Autodesk Fusion 360 part; units mm, degrees
(part 4 of 5)
  spline S14 degree 5 poles (-104.9129, -27.728) (-104.9107, -27.7405) (-104.9058, -27.7653) (-104.8975, -27.8023) (-104.8848, -27.8513) (-104.8664, -27.9119) (-104.8463, -27.9721) (-104.8251, -28.0321) (-104.8033, -28.0919) (-104.7812, -28.1516) (-104.7586, -28.2113) (-104.7355, -28.2708) (-104.7117, -28.3301) (-104.687, -28.3892) (-104.6615, -28.4481) (-104.6353, -28.5068) (-104.6083, -28.5653) (-104.5809, -28.6236) (-104.5529, -28.6818) (-104.5245, -28.7398) (-104.4956, -28.7977) (-104.4663, -28.8555) (-104.4364, -28.9131) (-104.4061, -28.9706) (-104.3752, -29.0279) (-104.3439, -29.085) (-104.312, -29.142) (-104.2798, -29.1989) (-104.2471, -29.2556) (-104.214, -29.3121) (-104.1805, -29.3686) (-104.1466, -29.4249) (-104.1123, -29.481) (-104.0776, -29.537) (-104.0425, -29.5929) (-104.0069, -29.6486) (-103.971, -29.7042) (-103.9348, -29.7596) (-103.8981, -29.8149) (-103.8611, -29.8701) (-103.8237, -29.9251) (-103.786, -29.98) (-103.7479, -30.0347) (-103.7094, -30.0893) (-103.6707, -30.1438) (-103.6315, -30.1981) (-103.592, -30.2523) (-103.5522, -30.3063) (-103.5121, -30.3603) (-103.4716, -30.414) (-103.4308, -30.4677) (-103.3896, -30.5212) (-103.3482, -30.5745) (-103.3064, -30.6277) (-103.2643, -30.6808) (-103.2219, -30.7337) (-103.1792, -30.7865) (-103.1362, -30.8392) (-103.0928, -30.8917) (-103.0492, -30.9441) (-103.0053, -30.9963) (-102.9611, -31.0484) (-102.9165, -31.1004) (-102.8717, -31.1522) (-102.8266, -31.2039) (-102.7812, -31.2554) (-102.7355, -31.3068) (-102.6896, -31.3581) (-102.6433, -31.4092) (-102.5968, -31.4601) (-102.55, -31.511) (-102.5123, -31.5515) (-102.4839, -31.5819) (-102.4649, -31.6021) (-102.4554, -31.6122) knots 0 0 0 0 0 0 0.01428571 0.02857143 0.04285714 0.05714286 0.07142857 0.08571429 0.1 0.11428571 0.12857143 0.14285714 0.15714286 0.17142857 0.18571429 0.2 0.21428571 0.22857143 0.24285714 0.25714286 0.27142857 0.28571429 0.3 0.31428571 0.32857143 0.34285714 0.35714286 0.37142857 0.38571429 0.4 0.41428571 0.42857143 0.44285714 0.45714286 0.47142857 0.48571429 0.5 0.51428571 0.52857143 0.54285714 0.55714286 0.57142857 0.58571429 0.6 0.61428571 0.62857143 0.64285714 0.65714286 0.67142857 0.68571429 0.7 0.71428571 0.72857143 0.74285714 0.75714286 0.77142857 0.78571429 0.8 0.81428571 0.82857143 0.84285714 0.85714286 0.87142857 0.88571429 0.9 0.91428571 0.92857143 0.94285714 0.95714286 0.97142857 0.98571429 1 1 1 1 1 1
  arc A30 (-102.4554, -31.6122) -> (-100.7277, -31.1492) centre (-110, 0) ccw
  spline S15 degree 5 poles (-100.7277, -31.1492) (-100.7245, -31.1357) (-100.7182, -31.1088) (-100.7088, -31.0683) (-100.6964, -31.0143) (-100.6813, -30.9469) (-100.6665, -30.8795) (-100.652, -30.8121) (-100.6378, -30.7447) (-100.624, -30.6774) (-100.6104, -30.61) (-100.5972, -30.5427) (-100.5843, -30.4755) (-100.5717, -30.4082) (-100.5594, -30.341) (-100.5475, -30.2738) (-100.5359, -30.2066) (-100.5247, -30.1394) (-100.5137, -30.0723) (-100.5031, -30.0052) (-100.4929, -29.9382) (-100.483, -29.8712) (-100.4734, -29.8042) (-100.4642, -29.7373) (-100.4553, -29.6704) (-100.4468, -29.6035) (-100.4386, -29.5367) (-100.4308, -29.47) (-100.4233, -29.4032) (-100.4162, -29.3366) (-100.4095, -29.27) (-100.4031, -29.2034) (-100.3971, -29.1369) (-100.3915, -29.0704) (-100.3863, -29.004) (-100.3814, -28.9377) (-100.3769, -28.8714) (-100.3728, -28.8052) (-100.3691, -28.739) (-100.3658, -28.673) (-100.3629, -28.607) (-100.3605, -28.541) (-100.3584, -28.4752) (-100.3568, -28.4094) (-100.3555, -28.3437) (-100.3547, -28.2781) (-100.3544, -28.2125) (-100.3544, -28.1471) (-100.3549, -28.0817) (-100.3559, -28.0164) (-100.3573, -27.9513) (-100.3592, -27.8862) (-100.3616, -27.8213) (-100.3646, -27.7565) (-100.3681, -27.6918) (-100.372, -27.6272) (-100.3765, -27.5627) (-100.3813, -27.4983) (-100.3867, -27.4341) (-100.3926, -27.37) (-100.3992, -27.306) (-100.4066, -27.2423) (-100.4148, -27.1788) (-100.4238, -27.1155) (-100.4335, -27.0524) (-100.4438, -26.9894) (-100.4545, -26.9266) (-100.4656, -26.8639) (-100.4772, -26.8014) (-100.4899, -26.7392) (-100.5043, -26.6775) (-100.5177, -26.6288) (-100.5291, -26.5926) (-100.5373, -26.5686) (-100.5415, -26.5567) knots -1 -1 -1 -1 -1 -1 -0.98571429 -0.97142857 -0.95714286 -0.94285714 -0.92857143 -0.91428571 -0.9 -0.88571429 -0.87142857 -0.85714286 -0.84285714 -0.82857143 -0.81428571 -0.8 -0.78571429 -0.77142857 -0.75714286 -0.74285714 -0.72857143 -0.71428571 -0.7 -0.68571429 -0.67142857 -0.65714286 -0.64285714 -0.62857143 -0.61428571 -0.6 -0.58571429 -0.57142857 -0.55714286 -0.54285714 -0.52857143 -0.51428571 -0.5 -0.48571429 -0.47142857 -0.45714286 -0.44285714 -0.42857143 -0.41428571 -0.4 -0.38571429 -0.37142857 -0.35714286 -0.34285714 -0.32857143 -0.31428571 -0.3 -0.28571429 -0.27142857 -0.25714286 -0.24285714 -0.22857143 -0.21428571 -0.2 -0.18571429 -0.17142857 -0.15714286 -0.14285714 -0.12857143 -0.11428571 -0.1 -0.08571429 -0.07142857 -0.05714286 -0.04285714 -0.02857143 -0.01428571 0 0 0 0 0 0
  line L15 (-100.5415, -26.5567) -> (-100.5754, -26.4615)
  arc A31 (-100.0022, -25.1964) -> (-100.5754, -26.4615) centre (-99.6334, -26.1259) ccw
  arc A32 (-100.0022, -25.1964) -> (-99.2529, -24.8861) centre (-110, 0) ccw
  arc A33 (-97.9531, -25.3753) -> (-99.2529, -24.8861) centre (-98.8565, -25.8041) ccw
  line L16 (-97.9531, -25.3753) -> (-97.9097, -25.4666)
  spline S16 degree 5 poles (-97.9097, -25.4666) (-97.9043, -25.478) (-97.8932, -25.5007) (-97.8756, -25.5344) (-97.8506, -25.5783) (-97.8172, -25.6321) (-97.7822, -25.6851) (-97.7462, -25.7375) (-97.7097, -25.7897) (-97.6728, -25.8417) (-97.6356, -25.8934) (-97.5979, -25.9449) (-97.5595, -25.9961) (-97.5204, -26.0468) (-97.4805, -26.0971) (-97.44, -26.1469) (-97.3988, -26.1965) (-97.3572, -26.2457) (-97.3151, -26.2946) (-97.2726, -26.3434) (-97.2298, -26.3918) (-97.1865, -26.44) (-97.1427, -26.488) (-97.0985, -26.5356) (-97.0539, -26.583) (-97.0088, -26.6301) (-96.9633, -26.6769) (-96.9175, -26.7234) (-96.8712, -26.7698) (-96.8246, -26.8158) (-96.7777, -26.8617) (-96.7303, -26.9073) (-96.6827, -26.9526) (-96.6346, -26.9977) (-96.5863, -27.0426) (-96.5375, -27.0872) (-96.4885, -27.1316) (-96.4391, -27.1758) (-96.3894, -27.2197) (-96.3393, -27.2634) (-96.289, -27.3069) (-96.2383, -27.3501) (-96.1874, -27.3931) (-96.1361, -27.4359) (-96.0845, -27.4785) (-96.0327, -27.5208) (-95.9805, -27.563) (-95.9281, -27.6049) (-95.8753, -27.6466) (-95.8223, -27.688) (-95.769, -27.7293) (-95.7154, -27.7703) (-95.6616, -27.8111) (-95.6074, -27.8517) (-95.5531, -27.892) (-95.4984, -27.9322) (-95.4435, -27.9721) (-95.3883, -28.0119) (-95.3328, -28.0514) (-95.2771, -28.0907) (-95.2212, -28.1298) (-95.165, -28.1687) (-95.1085, -28.2073) (-95.0518, -28.2458) (-94.9949, -28.284) (-94.9377, -28.322) (-94.8803, -28.3599) (-94.8226, -28.3975) (-94.7647, -28.4349) (-94.7065, -28.4721) (-94.6482, -28.509) (-94.6013, -28.5385) (-94.566, -28.5604) (-94.5425, -28.575) (-94.5307, -28.5823) knots 0 0 0 0 0 0 0.01428571 0.02857143 0.04285714 0.05714286 0.07142857 0.08571429 0.1 0.11428571 0.12857143 0.14285714 0.15714286 0.17142857 0.18571429 0.2 0.21428571 0.22857143 0.24285714 0.25714286 0.27142857 0.28571429 0.3 0.31428571 0.32857143 0.34285714 0.35714286 0.37142857 0.38571429 0.4 0.41428571 0.42857143 0.44285714 0.45714286 0.47142857 0.48571429 0.5 0.51428571 0.52857143 0.54285714 0.55714286 0.57142857 0.58571429 0.6 0.61428571 0.62857143 0.64285714 0.65714286 0.67142857 0.68571429 0.7 0.71428571 0.72857143 0.74285714 0.75714286 0.77142857 0.78571429 0.8 0.81428571 0.82857143 0.84285714 0.85714286 0.87142857 0.88571429 0.9 0.91428571 0.92857143 0.94285714 0.95714286 0.97142857 0.98571429 1 1 1 1 1 1
  arc A34 (-94.5307, -28.5823) -> (-92.9816, -27.688) centre (-110, 0) ccw
  spline S17 degree 5 poles (-92.9816, -27.688) (-92.9821, -27.6741) (-92.9829, -27.6464) (-92.9843, -27.6049) (-92.9864, -27.5496) (-92.9892, -27.4806) (-92.9923, -27.4116) (-92.9958, -27.3428) (-92.9995, -27.274) (-93.0035, -27.2054) (-93.0079, -27.1368) (-93.0125, -27.0684) (-93.0175, -27.0001) (-93.0227, -26.9318) (-93.0283, -26.8637) (-93.0342, -26.7957) (-93.0404, -26.7278) (-93.0469, -26.6601) (-93.0537, -26.5924) (-93.0608, -26.5249) (-93.0683, -26.4574) (-93.076, -26.3902) (-93.0841, -26.323) (-93.0925, -26.2559) (-93.1013, -26.189) (-93.1103, -26.1223) (-93.1197, -26.0556) (-93.1295, -25.9891) (-93.1395, -25.9227) (-93.1499, -25.8565) (-93.1607, -25.7904) (-93.1717, -25.7245) (-93.1832, -25.6587) (-93.1949, -25.593) (-93.2071, -25.5275) (-93.2195, -25.4622) (-93.2324, -25.397) (-93.2455, -25.332) (-93.2591, -25.2671) (-93.273, -25.2025) (-93.2873, -25.1379) (-93.302, -25.0736) (-93.317, -25.0095) (-93.3324, -24.9455) (-93.3483, -24.8817) (-93.3645, -24.8181) (-93.3811, -24.7547) (-93.3981, -24.6915) (-93.4155, -24.6285) (-93.4333, -24.5657) (-93.4515, -24.5031) (-93.4702, -24.4408) (-93.4894, -24.3787) (-93.509, -24.3169) (-93.5291, -24.2553) (-93.5497, -24.1939) (-93.5706, -24.1328) (-93.592, -24.0718) (-93.6138, -24.0112) (-93.6361, -23.9508) (-93.659, -23.8907) (-93.6826, -23.8311) (-93.707, -23.7718) (-93.7321, -23.713) (-93.7578, -23.6546) (-93.7841, -23.5965) (-93.8106, -23.5386) (-93.8375, -23.4809) (-93.865, -23.4235) (-93.8933, -23.3667) (-93.9232, -23.3108) (-93.9488, -23.2672) (-93.9691, -23.2352) (-93.9832, -23.2142) (-93.9904, -23.2037) knots -1 -1 -1 -1 -1 -1 -0.98571429 -0.97142857 -0.95714286 -0.94285714 -0.92857143 -0.91428571 -0.9 -0.88571429 -0.87142857 -0.85714286 -0.84285714 -0.82857143 -0.81428571 -0.8 -0.78571429 -0.77142857 -0.75714286 -0.74285714 -0.72857143 -0.71428571 -0.7 -0.68571429 -0.67142857 -0.65714286 -0.64285714 -0.62857143 -0.61428571 -0.6 -0.58571429 -0.57142857 -0.55714286 -0.54285714 -0.52857143 -0.51428571 -0.5 -0.48571429 -0.47142857 -0.45714286 -0.44285714 -0.42857143 -0.41428571 -0.4 -0.38571429 -0.37142857 -0.35714286 -0.34285714 -0.32857143 -0.31428571 -0.3 -0.28571429 -0.27142857 -0.25714286 -0.24285714 -0.22857143 -0.21428571 -0.2 -0.18571429 -0.17142857 -0.15714286 -0.14285714 -0.12857143 -0.11428571 -0.1 -0.08571429 -0.07142857 -0.05714286 -0.04285714 -0.02857143 -0.01428571 0 0 0 0 0 0
  line L17 (-93.9904, -23.2037) -> (-94.0478, -23.1206)
  arc A35 (-93.8216, -21.7503) -> (-94.0478, -23.1206) centre (-93.2247, -22.5527) ccw
  arc A36 (-93.8216, -21.7503) -> (-93.1781, -21.2566) centre (-110, 0) ccw
  arc A37 (-91.796, -21.3926) -> (-93.1781, -21.2566) centre (-92.5576, -22.0407) ccw
  line L18 (-91.796, -21.3926) -> (-91.7305, -21.4696)
  spline S18 degree 5 poles (-91.7305, -21.4696) (-91.7223, -21.4793) (-91.7056, -21.4983) (-91.68, -21.5263) (-91.6444, -21.5623) (-91.5982, -21.6056) (-91.5507, -21.6477) (-91.5024, -21.689) (-91.4536, -21.73) (-91.4046, -21.7706) (-91.3552, -21.811) (-91.3054, -21.851) (-91.2551, -21.8904) (-91.2042, -21.9293) (-91.1527, -21.9675) (-91.1006, -22.0052) (-91.0481, -22.0424) (-90.9951, -22.0792) (-90.9418, -22.1156) (-90.8881, -22.1516) (-90.8342, -22.1874) (-90.7799, -22.2227) (-90.7252, -22.2577) (-90.6702, -22.2923) (-90.6148, -22.3265) (-90.5591, -22.3603) (-90.5031, -22.3937) (-90.4467, -22.4268) (-90.3901, -22.4596) (-90.3331, -22.4921) (-90.2759, -22.5242) (-90.2184, -22.556) (-90.1606, -22.5875) (-90.1025, -22.6186) (-90.0442, -22.6494) (-89.9856, -22.6799) (-89.9267, -22.7101) (-89.8675, -22.74) (-89.8082, -22.7695) (-89.7485, -22.7988) (-89.6886, -22.8277) (-89.6285, -22.8564) (-89.5682, -22.8848) (-89.5076, -22.9128) (-89.4467, -22.9406) (-89.3857, -22.9681) (-89.3244, -22.9953) (-89.2629, -23.0222) (-89.2012, -23.0488) (-89.1392, -23.0751) (-89.077, -23.1011) (-89.0147, -23.1269) (-88.9521, -23.1524) (-88.8893, -23.1776) (-88.8263, -23.2025) (-88.7631, -23.2271) (-88.6997, -23.2515) (-88.6362, -23.2756) (-88.5724, -23.2994) (-88.5084, -23.323) (-88.4442, -23.3462) (-88.3799, -23.3693) (-88.3153, -23.392) (-88.2506, -23.4145) (-88.1857, -23.4367) (-88.1206, -23.4586) (-88.0554, -23.4803) (-87.9899, -23.5017) (-87.9243, -23.5228) (-87.8585, -23.5437) (-87.7926, -23.5643) (-87.7397, -23.5806) (-87.6999, -23.5927) (-87.6734, -23.6007) (-87.6601, -23.6047) knots 0 0 0 0 0 0 0.01428571 0.02857143 0.04285714 0.05714286 0.07142857 0.08571429 0.1 0.11428571 0.12857143 0.14285714 0.15714286 0.17142857 0.18571429 0.2 0.21428571 0.22857143 0.24285714 0.25714286 0.27142857 0.28571429 0.3 0.31428571 0.32857143 0.34285714 0.35714286 0.37142857 0.38571429 0.4 0.41428571 0.42857143 0.44285714 0.45714286 0.47142857 0.48571429 0.5 0.51428571 0.52857143 0.54285714 0.55714286 0.57142857 0.58571429 0.6 0.61428571 0.62857143 0.64285714 0.65714286 0.67142857 0.68571429 0.7 0.71428571 0.72857143 0.74285714 0.75714286 0.77142857 0.78571429 0.8 0.81428571 0.82857143 0.84285714 0.85714286 0.87142857 0.88571429 0.9 0.91428571 0.92857143 0.94285714 0.95714286 0.97142857 0.98571429 1 1 1 1 1 1
  arc A38 (-87.6601, -23.6047) -> (-86.3953, -22.3399) centre (-110, 0) ccw
  spline S19 degree 5 poles (-86.3953, -22.3399) (-86.3993, -22.3266) (-86.4073, -22.3001) (-86.4194, -22.2603) (-86.4357, -22.2074) (-86.4563, -22.1415) (-86.4772, -22.0757) (-86.4983, -22.0101) (-86.5197, -21.9446) (-86.5414, -21.8794) (-86.5633, -21.8143) (-86.5855, -21.7494) (-86.608, -21.6847) (-86.6307, -21.6201) (-86.6538, -21.5558) (-86.677, -21.4916) (-86.7006, -21.4276) (-86.7244, -21.3638) (-86.7485, -21.3003) (-86.7729, -21.2369) (-86.7975, -21.1737) (-86.8224, -21.1107) (-86.8476, -21.0479) (-86.8731, -20.9853) (-86.8989, -20.923) (-86.9249, -20.8608) (-86.9512, -20.7988) (-86.9778, -20.7371) (-87.0047, -20.6756) (-87.0319, -20.6143) (-87.0594, -20.5533) (-87.0872, -20.4924) (-87.1152, -20.4318) (-87.1436, -20.3715) (-87.1723, -20.3114) (-87.2012, -20.2515) (-87.2305, -20.1918) (-87.26, -20.1325) (-87.2899, -20.0733) (-87.3201, -20.0144) (-87.3506, -19.9558) (-87.3814, -19.8975) (-87.4125, -19.8394) (-87.444, -19.7816) (-87.4758, -19.7241) (-87.5079, -19.6669) (-87.5404, -19.6099) (-87.5732, -19.5533) (-87.6063, -19.4969) (-87.6397, -19.4409) (-87.6735, -19.3852) (-87.7077, -19.3298) (-87.7423, -19.2748) (-87.7773, -19.2201) (-87.8126, -19.1658) (-87.8484, -19.1119) (-87.8844, -19.0582) (-87.9208, -19.0049) (-87.9576, -18.9519) (-87.9948, -18.8994) (-88.0325, -18.8473) (-88.0707, -18.7958) (-88.1096, -18.7449) (-88.149, -18.6946) (-88.189, -18.6448) (-88.2294, -18.5954) (-88.27, -18.5464) (-88.311, -18.4976) (-88.3523, -18.4493) (-88.3944, -18.4018) (-88.4377, -18.3556) (-88.4737, -18.32) (-88.5017, -18.2944) (-88.5207, -18.2777) (-88.5304, -18.2695) knots -1 -1 -1 -1 -1 -1 -0.98571429 -0.97142857 -0.95714286 -0.94285714 -0.92857143 -0.91428571 -0.9 -0.88571429 -0.87142857 -0.85714286 -0.84285714 -0.82857143 -0.81428571 -0.8 -0.78571429 -0.77142857 -0.75714286 -0.74285714 -0.72857143 -0.71428571 -0.7 -0.68571429 -0.67142857 -0.65714286 -0.64285714 -0.62857143 -0.61428571 -0.6 -0.58571429 -0.57142857 -0.55714286 -0.54285714 -0.52857143 -0.51428571 -0.5 -0.48571429 -0.47142857 -0.45714286 -0.44285714 -0.42857143 -0.41428571 -0.4 -0.38571429 -0.37142857 -0.35714286 -0.34285714 -0.32857143 -0.31428571 -0.3 -0.28571429 -0.27142857 -0.25714286 -0.24285714 -0.22857143 -0.21428571 -0.2 -0.18571429 -0.17142857 -0.15714286 -0.14285714 -0.12857143 -0.11428571 -0.1 -0.08571429 -0.07142857 -0.05714286 -0.04285714 -0.02857143 -0.01428571 0 0 0 0 0 0
  line L19 (-88.5304, -18.2695) -> (-88.6074, -18.204)
  arc A39 (-88.7434, -16.8219) -> (-88.6074, -18.204) centre (-87.9593, -17.4424) ccw
  arc A40 (-88.7434, -16.8219) -> (-88.2497, -16.1784) centre (-110, 0) ccw
  arc A41 (-86.8794, -15.9522) -> (-88.2497, -16.1784) centre (-87.4473, -16.7753) ccw
  line L20 (-86.8794, -15.9522) -> (-86.7963, -16.0096)
  spline S20 degree 5 poles (-86.7963, -16.0096) (-86.7858, -16.0168) (-86.7648, -16.0309) (-86.7328, -16.0512) (-86.6892, -16.0768) (-86.6333, -16.1067) (-86.5765, -16.135) (-86.5191, -16.1625) (-86.4614, -16.1894) (-86.4035, -16.2159) (-86.3454, -16.2422) (-86.287, -16.2679) (-86.2282, -16.293) (-86.1689, -16.3174) (-86.1093, -16.341) (-86.0492, -16.3639) (-85.9888, -16.3862) (-85.9282, -16.408) (-85.8672, -16.4294) (-85.8061, -16.4503) (-85.7447, -16.4709) (-85.6831, -16.491) (-85.6213, -16.5106) (-85.5592, -16.5298) (-85.4969, -16.5485) (-85.4343, -16.5667) (-85.3715, -16.5845) (-85.3085, -16.6019) (-85.2453, -16.6189) (-85.1819, -16.6355) (-85.1183, -16.6517) (-85.0545, -16.6676) (-84.9905, -16.683) (-84.9264, -16.698) (-84.8621, -16.7127) (-84.7975, -16.727) (-84.7329, -16.7409) (-84.668, -16.7545) (-84.603, -16.7676) (-84.5378, -16.7805) (-84.4725, -16.7929) (-84.407, -16.8051) (-84.3413, -16.8168) (-84.2755, -16.8283) (-84.2096, -16.8393) (-84.1435, -16.8501) (-84.0773, -16.8605) (-84.0109, -16.8705) (-83.9444, -16.8803) (-83.8777, -16.8897) (-83.811, -16.8987) (-83.7441, -16.9075) (-83.677, -16.9159) (-83.6098, -16.924) (-83.5426, -16.9317) (-83.4751, -16.9392) (-83.4076, -16.9463) (-83.3399, -16.9531) (-83.2722, -16.9596) (-83.2043, -16.9658) (-83.1363, -16.9717) (-83.0682, -16.9773) (-82.9999, -16.9825) (-82.9316, -16.9875) (-82.8632, -16.9921) (-82.7946, -16.9965) (-82.726, -17.0005) (-82.6572, -17.0042) (-82.5884, -17.0077) (-82.5194, -17.0108) (-82.4504, -17.0136) (-82.3951, -17.0157) (-82.3536, -17.0171) (-82.3259, -17.0179) (-82.312, -17.0184) knots 0 0 0 0 0 0 0.01428571 0.02857143 0.04285714 0.05714286 0.07142857 0.08571429 0.1 0.11428571 0.12857143 0.14285714 0.15714286 0.17142857 0.18571429 0.2 0.21428571 0.22857143 0.24285714 0.25714286 0.27142857 0.28571429 0.3 0.31428571 0.32857143 0.34285714 0.35714286 0.37142857 0.38571429 0.4 0.41428571 0.42857143 0.44285714 0.45714286 0.47142857 0.48571429 0.5 0.51428571 0.52857143 0.54285714 0.55714286 0.57142857 0.58571429 0.6 0.61428571 0.62857143 0.64285714 0.65714286 0.67142857 0.68571429 0.7 0.71428571 0.72857143 0.74285714 0.75714286 0.77142857 0.78571429 0.8 0.81428571 0.82857143 0.84285714 0.85714286 0.87142857 0.88571429 0.9 0.91428571 0.92857143 0.94285714 0.95714286 0.97142857 0.98571429 1 1 1 1 1 1
  arc A42 (-82.312, -17.0184) -> (-81.4177, -15.4693) centre (-110, 0) ccw
  spline S21 degree 5 poles (-81.4177, -15.4693) (-81.425, -15.4575) (-81.4396, -15.434) (-81.4615, -15.3987) (-81.491, -15.3518) (-81.5279, -15.2935) (-81.5651, -15.2353) (-81.6025, -15.1774) (-81.6401, -15.1197) (-81.678, -15.0623) (-81.716, -15.0051) (-81.7542, -14.9482) (-81.7927, -14.8915) (-81.8313, -14.835) (-81.8702, -14.7788) (-81.9093, -14.7229) (-81.9486, -14.6672) (-81.9881, -14.6117) (-82.0279, -14.5565) (-82.0678, -14.5016) (-82.108, -14.4469) (-82.1483, -14.3926) (-82.1889, -14.3384) (-82.2297, -14.2846) (-82.2707, -14.231) (-82.312, -14.1777) (-82.3534, -14.1247) (-82.3951, -14.0719) (-82.437, -14.0195) (-82.4792, -13.9673) (-82.5215, -13.9155) (-82.5641, -13.8639) (-82.6069, -13.8126) (-82.6499, -13.7617) (-82.6931, -13.711) (-82.7366, -13.6607) (-82.7803, -13.6106) (-82.8242, -13.5609) (-82.8684, -13.5115) (-82.9128, -13.4625) (-82.9574, -13.4137) (-83.0023, -13.3654) (-83.0474, -13.3173) (-83.0927, -13.2697) (-83.1383, -13.2223) (-83.1842, -13.1754) (-83.2302, -13.1288) (-83.2766, -13.0825) (-83.3231, -13.0367) (-83.3699, -12.9912) (-83.417, -12.9461) (-83.4644, -12.9015) (-83.512, -12.8573) (-83.56, -12.8135) (-83.6082, -12.7702) (-83.6566, -12.7274) (-83.7054, -12.6849) (-83.7543, -12.6428) (-83.8035, -12.6012) (-83.8531, -12.56) (-83.9029, -12.5195) (-83.9532, -12.4796) (-84.0039, -12.4405) (-84.0551, -12.4021) (-84.1066, -12.3644) (-84.1583, -12.3272) (-84.2103, -12.2903) (-84.2625, -12.2538) (-84.3149, -12.2178) (-84.3679, -12.1828) (-84.4217, -12.1494) (-84.4656, -12.1244) (-84.4993, -12.1068) (-84.522, -12.0957) (-84.5334, -12.0903) knots -1 -1 -1 -1 -1 -1 -0.98571429 -0.97142857 -0.95714286 -0.94285714 -0.92857143 -0.91428571 -0.9 -0.88571429 -0.87142857 -0.85714286 -0.84285714 -0.82857143 -0.81428571 -0.8 -0.78571429 -0.77142857 -0.75714286 -0.74285714 -0.72857143 -0.71428571 -0.7 -0.68571429 -0.67142857 -0.65714286 -0.64285714 -0.62857143 -0.61428571 -0.6 -0.58571429 -0.57142857 -0.55714286 -0.54285714 -0.52857143 -0.51428571 -0.5 -0.48571429 -0.47142857 -0.45714286 -0.44285714 -0.42857143 -0.41428571 -0.4 -0.38571429 -0.37142857 -0.35714286 -0.34285714 -0.32857143 -0.31428571 -0.3 -0.28571429 -0.27142857 -0.25714286 -0.24285714 -0.22857143 -0.21428571 -0.2 -0.18571429 -0.17142857 -0.15714286 -0.14285714 -0.12857143 -0.11428571 -0.1 -0.08571429 -0.07142857 -0.05714286 -0.04285714 -0.02857143 -0.01428571 0 0 0 0 0 0
  line L21 (-84.5334, -12.0903) -> (-84.6247, -12.0469)
  arc A43 (-85.1139, -10.7471) -> (-84.6247, -12.0469) centre (-84.1959, -11.1435) ccw
  arc A44 (-85.1139, -10.7471) -> (-84.8036, -9.9978) centre (-110, 0) ccw
  arc A45 (-83.5385, -9.4246) -> (-84.8036, -9.9978) centre (-83.8741, -10.3666) ccw
  line L22 (-83.5385, -9.4246) -> (-83.4433, -9.4585)
  spline S22 degree 5 poles (-83.4433, -9.4585) (-83.4314, -9.4627) (-83.4074, -9.4709) (-83.3712, -9.4823) (-83.3225, -9.4957) (-83.2608, -9.5101) (-83.1986, -9.5228) (-83.1361, -9.5344) (-83.0734, -9.5455) (-83.0106, -9.5562) (-82.9476, -9.5665) (-82.8845, -9.5762) (-82.8212, -9.5852) (-82.7577, -9.5934) (-82.694, -9.6008) (-82.63, -9.6074) (-82.5659, -9.6133) (-82.5017, -9.6187) (-82.4373, -9.6235) (-82.3728, -9.628) (-82.3082, -9.6319) (-82.2435, -9.6354) (-82.1787, -9.6384) (-82.1138, -9.6408) (-82.0487, -9.6427) (-81.9836, -9.6441) (-81.9183, -9.6451) (-81.8529, -9.6456) (-81.7875, -9.6456) (-81.7219, -9.6453) (-81.6563, -9.6445) (-81.5906, -9.6432) (-81.5248, -9.6416) (-81.459, -9.6395) (-81.393, -9.6371) (-81.327, -9.6342) (-81.261, -9.6309) (-81.1948, -9.6272) (-81.1286, -9.6231) (-81.0623, -9.6186) (-80.996, -9.6137) (-80.9296, -9.6085) (-80.8631, -9.6029) (-80.7966, -9.5969) (-80.73, -9.5905) (-80.6634, -9.5838) (-80.5968, -9.5767) (-80.53, -9.5692) (-80.4633, -9.5614) (-80.3965, -9.5532) (-80.3296, -9.5447) (-80.2627, -9.5358) (-80.1958, -9.5266) (-80.1288, -9.517) (-80.0618, -9.5071) (-79.9948, -9.4969) (-79.9277, -9.4863) (-79.8606, -9.4753) (-79.7934, -9.4641) (-79.7262, -9.4525) (-79.659, -9.4406) (-79.5918, -9.4283) (-79.5245, -9.4157) (-79.4573, -9.4028) (-79.39, -9.3896) (-79.3226, -9.376) (-79.2553, -9.3622) (-79.1879, -9.348) (-79.1205, -9.3335) (-79.0531, -9.3187) (-78.9857, -9.3036) (-78.9317, -9.2912) (-78.8912, -9.2818) (-78.8643, -9.2755) (-78.8508, -9.2723) knots 0 0 0 0 0 0 0.01428571 0.02857143 0.04285714 0.05714286 0.07142857 0.08571429 0.1 0.11428571 0.12857143 0.14285714 0.15714286 0.17142857 0.18571429 0.2 0.21428571 0.22857143 0.24285714 0.25714286 0.27142857 0.28571429 0.3 0.31428571 0.32857143 0.34285714 0.35714286 0.37142857 0.38571429 0.4 0.41428571 0.42857143 0.44285714 0.45714286 0.47142857 0.48571429 0.5 0.51428571 0.52857143 0.54285714 0.55714286 0.57142857 0.58571429 0.6 0.61428571 0.62857143 0.64285714 0.65714286 0.67142857 0.68571429 0.7 0.71428571 0.72857143 0.74285714 0.75714286 0.77142857 0.78571429 0.8 0.81428571 0.82857143 0.84285714 0.85714286 0.87142857 0.88571429 0.9 0.91428571 0.92857143 0.94285714 0.95714286 0.97142857 0.98571429 1 1 1 1 1 1
  arc A46 (-78.8508, -9.2723) -> (-78.3878, -7.5446) centre (-110, 0) ccw
  spline S23 degree 5 poles (-78.3878, -7.5446) (-78.3979, -7.5351) (-78.4181, -7.5161) (-78.4485, -7.4877) (-78.489, -7.45) (-78.5399, -7.4032) (-78.5908, -7.3567) (-78.6419, -7.3104) (-78.6932, -7.2645) (-78.7446, -7.2188) (-78.7961, -7.1734) (-78.8478, -7.1283) (-78.8996, -7.0835) (-78.9516, -7.0389) (-79.0037, -6.9947) (-79.0559, -6.9508) (-79.1083, -6.9072) (-79.1608, -6.8638) (-79.2135, -6.8208) (-79.2663, -6.7781) (-79.3192, -6.7357) (-79.3723, -6.6936) (-79.4255, -6.6518) (-79.4788, -6.6104) (-79.5323, -6.5692) (-79.586, -6.5284) (-79.6397, -6.4879) (-79.6937, -6.4478) (-79.7477, -6.408) (-79.8019, -6.3685) (-79.8562, -6.3293) (-79.9107, -6.2906) (-79.9653, -6.2521) (-80.02, -6.214) (-80.0749, -6.1763) (-80.1299, -6.1389) (-80.1851, -6.1019) (-80.2404, -6.0652) (-80.2958, -6.029) (-80.3514, -5.9931) (-80.4071, -5.9575) (-80.463, -5.9224) (-80.519, -5.8877) (-80.5751, -5.8534) (-80.6314, -5.8195) (-80.6879, -5.786) (-80.7444, -5.7529) (-80.8011, -5.7202) (-80.858, -5.688) (-80.915, -5.6561) (-80.9721, -5.6248) (-81.0294, -5.5939) (-81.0869, -5.5636) (-81.1445, -5.5337) (-81.2023, -5.5044) (-81.2602, -5.4755) (-81.3182, -5.4471) (-81.3764, -5.4191) (-81.4347, -5.3917) (-81.4932, -5.3647) (-81.5519, -5.3385) (-81.6108, -5.313) (-81.6699, -5.2883) (-81.7292, -5.2645) (-81.7887, -5.2414) (-81.8484, -5.2188) (-81.9081, -5.1967) (-81.9679, -5.1749) (-82.0279, -5.1537) (-82.0881, -5.1336) (-82.1487, -5.1152) (-82.1977, -5.1025) (-82.2347, -5.0942) (-82.2595, -5.0893) (-82.272, -5.0871) knots -1 -1 -1 -1 -1 -1 -0.98571429 -0.97142857 -0.95714286 -0.94285714 -0.92857143 -0.91428571 -0.9 -0.88571429 -0.87142857 -0.85714286 -0.84285714 -0.82857143 -0.81428571 -0.8 -0.78571429 -0.77142857 -0.75714286 -0.74285714 -0.72857143 -0.71428571 -0.7 -0.68571429 -0.67142857 -0.65714286 -0.64285714 -0.62857143 -0.61428571 -0.6 -0.58571429 -0.57142857 -0.55714286 -0.54285714 -0.52857143 -0.51428571 -0.5 -0.48571429 -0.47142857 -0.45714286 -0.44285714 -0.42857143 -0.41428571 -0.4 -0.38571429 -0.37142857 -0.35714286 -0.34285714 -0.32857143 -0.31428571 -0.3 -0.28571429 -0.27142857 -0.25714286 -0.24285714 -0.22857143 -0.21428571 -0.2 -0.18571429 -0.17142857 -0.15714286 -0.14285714 -0.12857143 -0.11428571 -0.1 -0.08571429 -0.07142857 -0.05714286 -0.04285714 -0.02857143 -0.01428571 0 0 0 0 0 0
  line L23 (-82.272, -5.0871) -> (-82.3714, -5.0688)
  arc A47 (-83.1803, -3.9399) -> (-82.3714, -5.0688) centre (-82.191, -4.0852) ccw
  arc A48 (-83.1803, -3.9399) -> (-83.0745, -3.1358) centre (-110, 0) ccw
  arc A49 (-82.0009, -2.2547) -> (-83.0745, -3.1358) centre (-82.0812, -3.2515) ccw
  line L24 (-82.0009, -2.2547) -> (-81.9002, -2.2628)
  spline S24 degree 5 poles (-81.9002, -2.2628) (-81.8876, -2.2638) (-81.8623, -2.2655) (-81.8244, -2.2672) (-81.7738, -2.2675) (-81.7105, -2.2655) (-81.6472, -2.2616) (-81.5838, -2.2567) (-81.5203, -2.2511) (-81.4569, -2.2452) (-81.3934, -2.2388) (-81.33, -2.2319) (-81.2665, -2.2242) (-81.203, -2.2157) (-81.1395, -2.2063) (-81.0761, -2.1962) (-81.0126, -2.1853) (-80.9492, -2.1738) (-80.8857, -2.1619) (-80.8223, -2.1495) (-80.7589, -2.1366) (-80.6955, -2.1232) (-80.6321, -2.1093) (-80.5688, -2.0948) (-80.5054, -2.0798) (-80.4421, -2.0643) (-80.3788, -2.0484) (-80.3156, -2.0319) (-80.2523, -2.015) (-80.1891, -1.9977) (-80.1259, -1.98) (-80.0628, -1.9618) (-79.9997, -1.9432) (-79.9366, -1.9241) (-79.8736, -1.9047) (-79.8105, -1.8848) (-79.7476, -1.8645) (-79.6846, -1.8438) (-79.6217, -1.8227) (-79.5589, -1.8012) (-79.496, -1.7794) (-79.4333, -1.7571) (-79.3705, -1.7345) (-79.3078, -1.7115) (-79.2452, -1.6881) (-79.1826, -1.6644) (-79.12, -1.6402) (-79.0575, -1.6158) (-78.995, -1.5909) (-78.9326, -1.5658) (-78.8703, -1.5402) (-78.8079, -1.5143) (-78.7457, -1.4881) (-78.6835, -1.4615) (-78.6213, -1.4346) (-78.5592, -1.4073) (-78.4971, -1.3797) (-78.4351, -1.3518) (-78.3732, -1.3236) (-78.3113, -1.295) (-78.2495, -1.2661) (-78.1877, -1.2368) (-78.126, -1.2073) (-78.0644, -1.1774) (-78.0028, -1.1472) (-77.9412, -1.1167) (-77.8798, -1.0858) (-77.8184, -1.0547) (-77.757, -1.0233) (-77.6957, -0.9915) (-77.6345, -0.9594) (-77.5856, -0.9336) (-77.5489, -0.914) (-77.5245, -0.9009) (-77.5123, -0.8943) knots 0 0 0 0 0 0 0.01428571 0.02857143 0.04285714 0.05714286 0.07142857 0.08571429 0.1 0.11428571 0.12857143 0.14285714 0.15714286 0.17142857 0.18571429 0.2 0.21428571 0.22857143 0.24285714 0.25714286 0.27142857 0.28571429 0.3 0.31428571 0.32857143 0.34285714 0.35714286 0.37142857 0.38571429 0.4 0.41428571 0.42857143 0.44285714 0.45714286 0.47142857 0.48571429 0.5 0.51428571 0.52857143 0.54285714 0.55714286 0.57142857 0.58571429 0.6 0.61428571 0.62857143 0.64285714 0.65714286 0.67142857 0.68571429 0.7 0.71428571 0.72857143 0.74285714 0.75714286 0.77142857 0.78571429 0.8 0.81428571 0.82857143 0.84285714 0.85714286 0.87142857 0.88571429 0.9 0.91428571 0.92857143 0.94285714 0.95714286 0.97142857 0.98571429 1 1 1 1 1 1
  arc A50 (-77.5123, -0.8943) -> (-77.5123, 0.8943) centre (-110, 0) ccw
  spline S25 degree 5 poles (-77.5123, 0.8943) (-77.5245, 0.9009) (-77.5489, 0.914) (-77.5856, 0.9336) (-77.6345, 0.9594) (-77.6957, 0.9915) (-77.757, 1.0233) (-77.8184, 1.0547) (-77.8798, 1.0858) (-77.9412, 1.1167) (-78.0028, 1.1472) (-78.0644, 1.1774) (-78.126, 1.2073) (-78.1877, 1.2368) (-78.2495, 1.2661) (-78.3113, 1.295) (-78.3732, 1.3236) (-78.4351, 1.3518) (-78.4971, 1.3797) (-78.5592, 1.4073) (-78.6213, 1.4346) (-78.6835, 1.4615) (-78.7457, 1.4881) (-78.8079, 1.5143) (-78.8703, 1.5402) (-78.9326, 1.5658) (-78.995, 1.5909) (-79.0575, 1.6158) (-79.12, 1.6402) (-79.1826, 1.6644) (-79.2452, 1.6881) (-79.3078, 1.7115) (-79.3705, 1.7345) (-79.4333, 1.7571) (-79.496, 1.7794) (-79.5589, 1.8012) (-79.6217, 1.8227) (-79.6846, 1.8438) (-79.7476, 1.8645) (-79.8105, 1.8848) (-79.8736, 1.9047) (-79.9366, 1.9241) (-79.9997, 1.9432) (-80.0628, 1.9618) (-80.1259, 1.98) (-80.1891, 1.9977) (-80.2523, 2.015) (-80.3156, 2.0319) (-80.3788, 2.0484) (-80.4421, 2.0643) (-80.5054, 2.0798) (-80.5688, 2.0948) (-80.6321, 2.1093) (-80.6955, 2.1232) (-80.7589, 2.1366) (-80.8223, 2.1495) (-80.8857, 2.1619) (-80.9492, 2.1738) (-81.0126, 2.1853) (-81.0761, 2.1962) (-81.1395, 2.2063) (-81.203, 2.2157) (-81.2665, 2.2242) (-81.33, 2.2319) (-81.3934, 2.2388) (-81.4569, 2.2452) (-81.5203, 2.2511) (-81.5838, 2.2567) (-81.6472, 2.2616) (-81.7105, 2.2655) (-81.7738, 2.2675) (-81.8244, 2.2672) (-81.8623, 2.2655) (-81.8876, 2.2638) (-81.9002, 2.2628) knots -1 -1 -1 -1 -1 -1 -0.98571429 -0.97142857 -0.95714286 -0.94285714 -0.92857143 -0.91428571 -0.9 -0.88571429 -0.87142857 -0.85714286 -0.84285714 -0.82857143 -0.81428571 -0.8 -0.78571429 -0.77142857 -0.75714286 -0.74285714 -0.72857143 -0.71428571 -0.7 -0.68571429 -0.67142857 -0.65714286 -0.64285714 -0.62857143 -0.61428571 -0.6 -0.58571429 -0.57142857 -0.55714286 -0.54285714 -0.52857143 -0.51428571 -0.5 -0.48571429 -0.47142857 -0.45714286 -0.44285714 -0.42857143 -0.41428571 -0.4 -0.38571429 -0.37142857 -0.35714286 -0.34285714 -0.32857143 -0.31428571 -0.3 -0.28571429 -0.27142857 -0.25714286 -0.24285714 -0.22857143 -0.21428571 -0.2 -0.18571429 -0.17142857 -0.15714286 -0.14285714 -0.12857143 -0.11428571 -0.1 -0.08571429 -0.07142857 -0.05714286 -0.04285714 -0.02857143 -0.01428571 0 0 0 0 0 0
  line L25 (-81.9002, 2.2628) -> (-82.0009, 2.2547)
  arc A51 (-83.0745, 3.1358) -> (-82.0009, 2.2547) centre (-82.0812, 3.2515) ccw
  arc A52 (-83.0745, 3.1358) -> (-83.1803, 3.9399) centre (-110, 0) ccw
  arc A53 (-82.3714, 5.0688) -> (-83.1803, 3.9399) centre (-82.191, 4.0852) ccw
  line L26 (-82.3714, 5.0688) -> (-82.272, 5.0871)
  spline S26 degree 5 poles (-82.272, 5.0871) (-82.2595, 5.0893) (-82.2347, 5.0942) (-82.1977, 5.1025) (-82.1487, 5.1152) (-82.0881, 5.1336) (-82.0279, 5.1537) (-81.9679, 5.1749) (-81.9081, 5.1967) (-81.8484, 5.2188) (-81.7887, 5.2414) (-81.7292, 5.2645) (-81.6699, 5.2883) (-81.6108, 5.313) (-81.5519, 5.3385) (-81.4932, 5.3647) (-81.4347, 5.3917) (-81.3764, 5.4191) (-81.3182, 5.4471) (-81.2602, 5.4755) (-81.2023, 5.5044) (-81.1445, 5.5337) (-81.0869, 5.5636) (-81.0294, 5.5939) (-80.9721, 5.6248) (-80.915, 5.6561) (-80.858, 5.688) (-80.8011, 5.7202) (-80.7444, 5.7529) (-80.6879, 5.786) (-80.6314, 5.8195) (-80.5751, 5.8534) (-80.519, 5.8877) (-80.463, 5.9224) (-80.4071, 5.9575) (-80.3514, 5.9931) (-80.2958, 6.029) (-80.2404, 6.0652) (-80.1851, 6.1019) (-80.1299, 6.1389) (-80.0749, 6.1763) (-80.02, 6.214) (-79.9653, 6.2521) (-79.9107, 6.2906) (-79.8562, 6.3293) (-79.8019, 6.3685) (-79.7477, 6.408) (-79.6937, 6.4478) (-79.6397, 6.4879) (-79.586, 6.5284) (-79.5323, 6.5692) (-79.4788, 6.6104) (-79.4255, 6.6518) (-79.3723, 6.6936) (-79.3192, 6.7357) (-79.2663, 6.7781) (-79.2135, 6.8208) (-79.1608, 6.8638) (-79.1083, 6.9072) (-79.0559, 6.9508) (-79.0037, 6.9947) (-78.9516, 7.0389) (-78.8996, 7.0835) (-78.8478, 7.1283) (-78.7961, 7.1734) (-78.7446, 7.2188) (-78.6932, 7.2645) (-78.6419, 7.3104) (-78.5908, 7.3567) (-78.5399, 7.4032) (-78.489, 7.45) (-78.4485, 7.4877) (-78.4181, 7.5161) (-78.3979, 7.5351) (-78.3878, 7.5446) knots 0 0 0 0 0 0 0.01428571 0.02857143 0.04285714 0.05714286 0.07142857 0.08571429 0.1 0.11428571 0.12857143 0.14285714 0.15714286 0.17142857 0.18571429 0.2 0.21428571 0.22857143 0.24285714 0.25714286 0.27142857 0.28571429 0.3 0.31428571 0.32857143 0.34285714 0.35714286 0.37142857 0.38571429 0.4 0.41428571 0.42857143 0.44285714 0.45714286 0.47142857 0.48571429 0.5 0.51428571 0.52857143 0.54285714 0.55714286 0.57142857 0.58571429 0.6 0.61428571 0.62857143 0.64285714 0.65714286 0.67142857 0.68571429 0.7 0.71428571 0.72857143 0.74285714 0.75714286 0.77142857 0.78571429 0.8 0.81428571 0.82857143 0.84285714 0.85714286 0.87142857 0.88571429 0.9 0.91428571 0.92857143 0.94285714 0.95714286 0.97142857 0.98571429 1 1 1 1 1 1
  arc A54 (-78.3878, 7.5446) -> (-78.8508, 9.2723) centre (-110, 0) ccw
  spline S27 degree 5 poles (-78.8508, 9.2723) (-78.8643, 9.2755) (-78.8912, 9.2818) (-78.9317, 9.2912) (-78.9857, 9.3036) (-79.0531, 9.3187) (-79.1205, 9.3335) (-79.1879, 9.348) (-79.2553, 9.3622) (-79.3226, 9.376) (-79.39, 9.3896) (-79.4573, 9.4028) (-79.5245, 9.4157) (-79.5918, 9.4283) (-79.659, 9.4406) (-79.7262, 9.4525) (-79.7934, 9.4641) (-79.8606, 9.4753) (-79.9277, 9.4863) (-79.9948, 9.4969) (-80.0618, 9.5071) (-80.1288, 9.517) (-80.1958, 9.5266) (-80.2627, 9.5358) (-80.3296, 9.5447) (-80.3965, 9.5532) (-80.4633, 9.5614) (-80.53, 9.5692) (-80.5968, 9.5767) (-80.6634, 9.5838) (-80.73, 9.5905) (-80.7966, 9.5969) (-80.8631, 9.6029) (-80.9296, 9.6085) (-80.996, 9.6137) (-81.0623, 9.6186) (-81.1286, 9.6231) (-81.1948, 9.6272) (-81.261, 9.6309) (-81.327, 9.6342) (-81.393, 9.6371) (-81.459, 9.6395) (-81.5248, 9.6416) (-81.5906, 9.6432) (-81.6563, 9.6445) (-81.7219, 9.6453) (-81.7875, 9.6456) (-81.8529, 9.6456) (-81.9183, 9.6451) (-81.9836, 9.6441) (-82.0487, 9.6427) (-82.1138, 9.6408) (-82.1787, 9.6384) (-82.2435, 9.6354) (-82.3082, 9.6319) (-82.3728, 9.628) (-82.4373, 9.6235) (-82.5017, 9.6187) (-82.5659, 9.6133) (-82.63, 9.6074) (-82.694, 9.6008) (-82.7577, 9.5934) (-82.8212, 9.5852) (-82.8845, 9.5762) (-82.9476, 9.5665) (-83.0106, 9.5562) (-83.0734, 9.5455) (-83.1361, 9.5344) (-83.1986, 9.5228) (-83.2608, 9.5101) (-83.3225, 9.4957) (-83.3712, 9.4823) (-83.4074, 9.4709) (-83.4314, 9.4627) (-83.4433, 9.4585) knots -1 -1 -1 -1 -1 -1 -0.98571429 -0.97142857 -0.95714286 -0.94285714 -0.92857143 -0.91428571 -0.9 -0.88571429 -0.87142857 -0.85714286 -0.84285714 -0.82857143 -0.81428571 -0.8 -0.78571429 -0.77142857 -0.75714286 -0.74285714 -0.72857143 -0.71428571 -0.7 -0.68571429 -0.67142857 -0.65714286 -0.64285714 -0.62857143 -0.61428571 -0.6 -0.58571429 -0.57142857 -0.55714286 -0.54285714 -0.52857143 -0.51428571 -0.5 -0.48571429 -0.47142857 -0.45714286 -0.44285714 -0.42857143 -0.41428571 -0.4 -0.38571429 -0.37142857 -0.35714286 -0.34285714 -0.32857143 -0.31428571 -0.3 -0.28571429 -0.27142857 -0.25714286 -0.24285714 -0.22857143 -0.21428571 -0.2 -0.18571429 -0.17142857 -0.15714286 -0.14285714 -0.12857143 -0.11428571 -0.1 -0.08571429 -0.07142857 -0.05714286 -0.04285714 -0.02857143 -0.01428571 0 0 0 0 0 0
  line L27 (-83.4433, 9.4585) -> (-83.5385, 9.4246)
  arc A55 (-84.8036, 9.9978) -> (-83.5385, 9.4246) centre (-83.8741, 10.3666) ccw
  arc A56 (-84.8036, 9.9978) -> (-85.1139, 10.7471) centre (-110, 0) ccw
  arc A57 (-84.6247, 12.0469) -> (-85.1139, 10.7471) centre (-84.1959, 11.1435) ccw
  line L28 (-84.6247, 12.0469) -> (-84.5334, 12.0903)
  spline S28 degree 5 poles (-84.5334, 12.0903) (-84.522, 12.0957) (-84.4993, 12.1068) (-84.4656, 12.1244) (-84.4217, 12.1494) (-84.3679, 12.1828) (-84.3149, 12.2178) (-84.2625, 12.2538) (-84.2103, 12.2903) (-84.1583, 12.3272) (-84.1066, 12.3644) (-84.0551, 12.4021) (-84.0039, 12.4405) (-83.9532, 12.4796) (-83.9029, 12.5195) (-83.8531, 12.56) (-83.8035, 12.6012) (-83.7543, 12.6428) (-83.7054, 12.6849) (-83.6566, 12.7274) (-83.6082, 12.7702) (-83.56, 12.8135) (-83.512, 12.8573) (-83.4644, 12.9015) (-83.417, 12.9461) (-83.3699, 12.9912) (-83.3231, 13.0367) (-83.2766, 13.0825) (-83.2302, 13.1288) (-83.1842, 13.1754) (-83.1383, 13.2223) (-83.0927, 13.2697) (-83.0474, 13.3173) (-83.0023, 13.3654) (-82.9574, 13.4137) (-82.9128, 13.4625) (-82.8684, 13.5115) (-82.8242, 13.5609) (-82.7803, 13.6106) (-82.7366, 13.6607) (-82.6931, 13.711) (-82.6499, 13.7617) (-82.6069, 13.8126) (-82.5641, 13.8639) (-82.5215, 13.9155) (-82.4792, 13.9673) (-82.437, 14.0195) (-82.3951, 14.0719) (-82.3534, 14.1247) (-82.312, 14.1777) (-82.2707, 14.231) (-82.2297, 14.2846) (-82.1889, 14.3384) (-82.1483, 14.3926) (-82.108, 14.4469) (-82.0678, 14.5016) (-82.0279, 14.5565) (-81.9881, 14.6117) (-81.9486, 14.6672) (-81.9093, 14.7229) (-81.8702, 14.7788) (-81.8313, 14.835) (-81.7927, 14.8915) (-81.7542, 14.9482) (-81.716, 15.0051) (-81.678, 15.0623) (-81.6401, 15.1197) (-81.6025, 15.1774) (-81.5651, 15.2353) (-81.5279, 15.2935) (-81.491, 15.3518) (-81.4615, 15.3987) (-81.4396, 15.434) (-81.425, 15.4575) (-81.4177, 15.4693) knots 0 0 0 0 0 0 0.01428571 0.02857143 0.04285714 0.05714286 0.07142857 0.08571429 0.1 0.11428571 0.12857143 0.14285714 0.15714286 0.17142857 0.18571429 0.2 0.21428571 0.22857143 0.24285714 0.25714286 0.27142857 0.28571429 0.3 0.31428571 0.32857143 0.34285714 0.35714286 0.37142857 0.38571429 0.4 0.41428571 0.42857143 0.44285714 0.45714286 0.47142857 0.48571429 0.5 0.51428571 0.52857143 0.54285714 0.55714286 0.57142857 0.58571429 0.6 0.61428571 0.62857143 0.64285714 0.65714286 0.67142857 0.68571429 0.7 0.71428571 0.72857143 0.74285714 0.75714286 0.77142857 0.78571429 0.8 0.81428571 0.82857143 0.84285714 0.85714286 0.87142857 0.88571429 0.9 0.91428571 0.92857143 0.94285714 0.95714286 0.97142857 0.98571429 1 1 1 1 1 1
  arc A58 (-81.4177, 15.4693) -> (-82.312, 17.0184) centre (-110, 0) ccw
  spline S29 degree 5 poles (-82.312, 17.0184) (-82.3259, 17.0179) (-82.3536, 17.0171) (-82.3951, 17.0157) (-82.4504, 17.0136) (-82.5194, 17.0108) (-82.5884, 17.0077) (-82.6572, 17.0042) (-82.726, 17.0005) (-82.7946, 16.9965) (-82.8632, 16.9921) (-82.9316, 16.9875) (-82.9999, 16.9825) (-83.0682, 16.9773) (-83.1363, 16.9717) (-83.2043, 16.9658) (-83.2722, 16.9596) (-83.3399, 16.9531) (-83.4076, 16.9463) (-83.4751, 16.9392) (-83.5426, 16.9317) (-83.6098, 16.924) (-83.677, 16.9159) (-83.7441, 16.9075) (-83.811, 16.8987) (-83.8777, 16.8897) (-83.9444, 16.8803) (-84.0109, 16.8705) (-84.0773, 16.8605) (-84.1435, 16.8501) (-84.2096, 16.8393) (-84.2755, 16.8283) (-84.3413, 16.8168) (-84.407, 16.8051) (-84.4725, 16.7929) (-84.5378, 16.7805) (-84.603, 16.7676) (-84.668, 16.7545) (-84.7329, 16.7409) (-84.7975, 16.727) (-84.8621, 16.7127) (-84.9264, 16.698) (-84.9905, 16.683) (-85.0545, 16.6676) (-85.1183, 16.6517) (-85.1819, 16.6355) (-85.2453, 16.6189) (-85.3085, 16.6019) (-85.3715, 16.5845) (-85.4343, 16.5667) (-85.4969, 16.5485) (-85.5592, 16.5298) (-85.6213, 16.5106) (-85.6831, 16.491) (-85.7447, 16.4709) (-85.8061, 16.4503) (-85.8672, 16.4294) (-85.9282, 16.408) (-85.9888, 16.3862) (-86.0492, 16.3639) (-86.1093, 16.341) (-86.1689, 16.3174) (-86.2282, 16.293) (-86.287, 16.2679) (-86.3454, 16.2422) (-86.4035, 16.2159) (-86.4614, 16.1894) (-86.5191, 16.1625) (-86.5765, 16.135) (-86.6333, 16.1067) (-86.6892, 16.0768) (-86.7328, 16.0512) (-86.7648, 16.0309) (-86.7858, 16.0168) (-86.7963, 16.0096) knots -1 -1 -1 -1 -1 -1 -0.98571429 -0.97142857 -0.95714286 -0.94285714 -0.92857143 -0.91428571 -0.9 -0.88571429 -0.87142857 -0.85714286 -0.84285714 -0.82857143 -0.81428571 -0.8 -0.78571429 -0.77142857 -0.75714286 -0.74285714 -0.72857143 -0.71428571 -0.7 -0.68571429 -0.67142857 -0.65714286 -0.64285714 -0.62857143 -0.61428571 -0.6 -0.58571429 -0.57142857 -0.55714286 -0.54285714 -0.52857143 -0.51428571 -0.5 -0.48571429 -0.47142857 -0.45714286 -0.44285714 -0.42857143 -0.41428571 -0.4 -0.38571429 -0.37142857 -0.35714286 -0.34285714 -0.32857143 -0.31428571 -0.3 -0.28571429 -0.27142857 -0.25714286 -0.24285714 -0.22857143 -0.21428571 -0.2 -0.18571429 -0.17142857 -0.15714286 -0.14285714 -0.12857143 -0.11428571 -0.1 -0.08571429 -0.07142857 -0.05714286 -0.04285714 -0.02857143 -0.01428571 0 0 0 0 0 0
  line L29 (-86.7963, 16.0096) -> (-86.8794, 15.9522)
  arc A59 (-88.2497, 16.1784) -> (-86.8794, 15.9522) centre (-87.4473, 16.7753) ccw
  arc A60 (-88.2497, 16.1784) -> (-88.7434, 16.8219) centre (-110, 0) ccw
  arc A61 (-88.6074, 18.204) -> (-88.7434, 16.8219) centre (-87.9593, 17.4424) ccw
  line L30 (-88.6074, 18.204) -> (-88.5304, 18.2695)
  spline S30 degree 5 poles (-88.5304, 18.2695) (-88.5207, 18.2777) (-88.5017, 18.2944) (-88.4737, 18.32) (-88.4377, 18.3556) (-88.3944, 18.4018) (-88.3523, 18.4493) (-88.311, 18.4976) (-88.27, 18.5464) (-88.2294, 18.5954) (-88.189, 18.6448) (-88.149, 18.6946) (-88.1096, 18.7449) (-88.0707, 18.7958) (-88.0325, 18.8473) (-87.9948, 18.8994) (-87.9576, 18.9519) (-87.9208, 19.0049) (-87.8844, 19.0582) (-87.8484, 19.1119) (-87.8126, 19.1658) (-87.7773, 19.2201) (-87.7423, 19.2748) (-87.7077, 19.3298) (-87.6735, 19.3852) (-87.6397, 19.4409) (-87.6063, 19.4969) (-87.5732, 19.5533) (-87.5404, 19.6099) (-87.5079, 19.6669) (-87.4758, 19.7241) (-87.444, 19.7816) (-87.4125, 19.8394) (-87.3814, 19.8975) (-87.3506, 19.9558) (-87.3201, 20.0144) (-87.2899, 20.0733) (-87.26, 20.1325) (-87.2305, 20.1918) (-87.2012, 20.2515) (-87.1723, 20.3114) (-87.1436, 20.3715) (-87.1152, 20.4318) (-87.0872, 20.4924) (-87.0594, 20.5533) (-87.0319, 20.6143) (-87.0047, 20.6756) (-86.9778, 20.7371) (-86.9512, 20.7988) (-86.9249, 20.8608) (-86.8989, 20.923) (-86.8731, 20.9853) (-86.8476, 21.0479) (-86.8224, 21.1107) (-86.7975, 21.1737) (-86.7729, 21.2369) (-86.7485, 21.3003) (-86.7244, 21.3638) (-86.7006, 21.4276) (-86.677, 21.4916) (-86.6538, 21.5558) (-86.6307, 21.6201) (-86.608, 21.6847) (-86.5855, 21.7494) (-86.5633, 21.8143) (-86.5414, 21.8794) (-86.5197, 21.9446) (-86.4983, 22.0101) (-86.4772, 22.0757) (-86.4563, 22.1415) (-86.4357, 22.2074) (-86.4194, 22.2603) (-86.4073, 22.3001) (-86.3993, 22.3266) (-86.3953, 22.3399) knots 0 0 0 0 0 0 0.01428571 0.02857143 0.04285714 0.05714286 0.07142857 0.08571429 0.1 0.11428571 0.12857143 0.14285714 0.15714286 0.17142857 0.18571429 0.2 0.21428571 0.22857143 0.24285714 0.25714286 0.27142857 0.28571429 0.3 0.31428571 0.32857143 0.34285714 0.35714286 0.37142857 0.38571429 0.4 0.41428571 0.42857143 0.44285714 0.45714286 0.47142857 0.48571429 0.5 0.51428571 0.52857143 0.54285714 0.55714286 0.57142857 0.58571429 0.6 0.61428571 0.62857143 0.64285714 0.65714286 0.67142857 0.68571429 0.7 0.71428571 0.72857143 0.74285714 0.75714286 0.77142857 0.78571429 0.8 0.81428571 0.82857143 0.84285714 0.85714286 0.87142857 0.88571429 0.9 0.91428571 0.92857143 0.94285714 0.95714286 0.97142857 0.98571429 1 1 1 1 1 1
  arc A62 (-86.3953, 22.3399) -> (-87.6601, 23.6047) centre (-110, 0) ccw
  spline S31 degree 5 poles (-87.6601, 23.6047) (-87.6734, 23.6007) (-87.6999, 23.5927) (-87.7397, 23.5806) (-87.7926, 23.5643) (-87.8585, 23.5437) (-87.9243, 23.5228) (-87.9899, 23.5017) (-88.0554, 23.4803) (-88.1206, 23.4586) (-88.1857, 23.4367) (-88.2506, 23.4145) (-88.3153, 23.392) (-88.3799, 23.3693) (-88.4442, 23.3462) (-88.5084, 23.323) (-88.5724, 23.2994) (-88.6362, 23.2756) (-88.6997, 23.2515) (-88.7631, 23.2271) (-88.8263, 23.2025) (-88.8893, 23.1776) (-88.9521, 23.1524) (-89.0147, 23.1269) (-89.077, 23.1011) (-89.1392, 23.0751) (-89.2012, 23.0488) (-89.2629, 23.0222) (-89.3244, 22.9953) (-89.3857, 22.9681) (-89.4467, 22.9406) (-89.5076, 22.9128) (-89.5682, 22.8848) (-89.6285, 22.8564) (-89.6886, 22.8277) (-89.7485, 22.7988) (-89.8082, 22.7695) (-89.8675, 22.74) (-89.9267, 22.7101) (-89.9856, 22.6799) (-90.0442, 22.6494) (-90.1025, 22.6186) (-90.1606, 22.5875) (-90.2184, 22.556) (-90.2759, 22.5242) (-90.3331, 22.4921) (-90.3901, 22.4596) (-90.4467, 22.4268) (-90.5031, 22.3937) (-90.5591, 22.3603) (-90.6148, 22.3265) (-90.6702, 22.2923) (-90.7252, 22.2577) (-90.7799, 22.2227) (-90.8342, 22.1874) (-90.8881, 22.1516) (-90.9418, 22.1156) (-90.9951, 22.0792) (-91.0481, 22.0424) (-91.1006, 22.0052) (-91.1527, 21.9675) (-91.2042, 21.9293) (-91.2551, 21.8904) (-91.3054, 21.851) (-91.3552, 21.811) (-91.4046, 21.7706) (-91.4536, 21.73) (-91.5024, 21.689) (-91.5507, 21.6477) (-91.5982, 21.6056) (-91.6444, 21.5623) (-91.68, 21.5263) (-91.7056, 21.4983) (-91.7223, 21.4793) (-91.7305, 21.4696) knots -1 -1 -1 -1 -1 -1 -0.98571429 -0.97142857 -0.95714286 -0.94285714 -0.92857143 -0.91428571 -0.9 -0.88571429 -0.87142857 -0.85714286 -0.84285714 -0.82857143 -0.81428571 -0.8 -0.78571429 -0.77142857 -0.75714286 -0.74285714 -0.72857143 -0.71428571 -0.7 -0.68571429 -0.67142857 -0.65714286 -0.64285714 -0.62857143 -0.61428571 -0.6 -0.58571429 -0.57142857 -0.55714286 -0.54285714 -0.52857143 -0.51428571 -0.5 -0.48571429 -0.47142857 -0.45714286 -0.44285714 -0.42857143 -0.41428571 -0.4 -0.38571429 -0.37142857 -0.35714286 -0.34285714 -0.32857143 -0.31428571 -0.3 -0.28571429 -0.27142857 -0.25714286 -0.24285714 -0.22857143 -0.21428571 -0.2 -0.18571429 -0.17142857 -0.15714286 -0.14285714 -0.12857143 -0.11428571 -0.1 -0.08571429 -0.07142857 -0.05714286 -0.04285714 -0.02857143 -0.01428571 0 0 0 0 0 0
  line L31 (-91.7305, 21.4696) -> (-91.796, 21.3926)
  arc A63 (-93.1781, 21.2566) -> (-91.796, 21.3926) centre (-92.5576, 22.0407) ccw
  arc A64 (-93.1781, 21.2566) -> (-93.8216, 21.7503) centre (-110, 0) ccw
  arc A65 (-94.0478, 23.1206) -> (-93.8216, 21.7503) centre (-93.2247, 22.5527) ccw
  line L32 (-94.0478, 23.1206) -> (-93.9904, 23.2037)
  spline S32 degree 5 poles (-93.9904, 23.2037) (-93.9832, 23.2142) (-93.9691, 23.2352) (-93.9488, 23.2672) (-93.9232, 23.3108) (-93.8933, 23.3667) (-93.865, 23.4235) (-93.8375, 23.4809) (-93.8106, 23.5386) (-93.7841, 23.5965) (-93.7578, 23.6546) (-93.7321, 23.713) (-93.707, 23.7718) (-93.6826, 23.8311) (-93.659, 23.8907) (-93.6361, 23.9508) (-93.6138, 24.0112) (-93.592, 24.0718) (-93.5706, 24.1328) (-93.5497, 24.1939) (-93.5291, 24.2553) (-93.509, 24.3169) (-93.4894, 24.3787) (-93.4702, 24.4408) (-93.4515, 24.5031) (-93.4333, 24.5657) (-93.4155, 24.6285) (-93.3981, 24.6915) (-93.3811, 24.7547) (-93.3645, 24.8181) (-93.3483, 24.8817) (-93.3324, 24.9455) (-93.317, 25.0095) (-93.302, 25.0736) (-93.2873, 25.1379) (-93.273, 25.2025) (-93.2591, 25.2671) (-93.2455, 25.332) (-93.2324, 25.397) (-93.2195, 25.4622) (-93.2071, 25.5275) (-93.1949, 25.593) (-93.1832, 25.6587) (-93.1717, 25.7245) (-93.1607, 25.7904) (-93.1499, 25.8565) (-93.1395, 25.9227) (-93.1295, 25.9891) (-93.1197, 26.0556) (-93.1103, 26.1223) (-93.1013, 26.189) (-93.0925, 26.2559) (-93.0841, 26.323) (-93.076, 26.3902) (-93.0683, 26.4574) (-93.0608, 26.5249) (-93.0537, 26.5924) (-93.0469, 26.6601) (-93.0404, 26.7278) (-93.0342, 26.7957) (-93.0283, 26.8637) (-93.0227, 26.9318) (-93.0175, 27.0001) (-93.0125, 27.0684) (-93.0079, 27.1368) (-93.0035, 27.2054) (-92.9995, 27.274) (-92.9958, 27.3428) (-92.9923, 27.4116) (-92.9892, 27.4806) (-92.9864, 27.5496) (-92.9843, 27.6049) (-92.9829, 27.6464) (-92.9821, 27.6741) (-92.9816, 27.688) knots 0 0 0 0 0 0 0.01428571 0.02857143 0.04285714 0.05714286 0.07142857 0.08571429 0.1 0.11428571 0.12857143 0.14285714 0.15714286 0.17142857 0.18571429 0.2 0.21428571 0.22857143 0.24285714 0.25714286 0.27142857 0.28571429 0.3 0.31428571 0.32857143 0.34285714 0.35714286 0.37142857 0.38571429 0.4 0.41428571 0.42857143 0.44285714 0.45714286 0.47142857 0.48571429 0.5 0.51428571 0.52857143 0.54285714 0.55714286 0.57142857 0.58571429 0.6 0.61428571 0.62857143 0.64285714 0.65714286 0.67142857 0.68571429 0.7 0.71428571 0.72857143 0.74285714 0.75714286 0.77142857 0.78571429 0.8 0.81428571 0.82857143 0.84285714 0.85714286 0.87142857 0.88571429 0.9 0.91428571 0.92857143 0.94285714 0.95714286 0.97142857 0.98571429 1 1 1 1 1 1
  arc A66 (-92.9816, 27.688) -> (-94.5307, 28.5823) centre (-110, 0) ccw